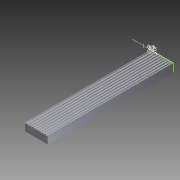
# Autodesk Inventor part: ruber2
Saved by Autodesk Inventor 2012 (Build 160160000, 160)
## iProperties
Created: 2013-08-22
Part Number: ruber2
Material: Default
Document SubType Name: Modeling
Designer: Dantro
Density: 1 g/cm^3
Author: Dantro
Autodesk Inventor part; units mm, degrees
ref_plane "YZ Plane" through (0, 0, 0) normal (1, 0, 0) x (0, 1, 0)
ref_plane "XZ Plane" through (0, 0, 0) normal (0, 1, 0) x (-1, 0, 0)
ref_plane "XY Plane" through (0, 0, 0) normal (0, 0, 1) x (1, 0, 0)
sketch "Sketch1" plane through (0, 0, 0) normal (0, 0, 1) x (1, 0, 0)
  line L0 (0, 0) -> (9, 0)
  line L1 (0.25, 3) -> (0, 3)
  line L2 (0.75, 3) -> (0.75, 2.7)
  line L3 (0.75, 2.7) -> (0.25, 2.7)
  line L4 (0.25, 2.7) -> (0.25, 3)
  line L5 (0.75, 3) -> (1, 3)
  line L6 (1.25, 3) -> (1, 3)
  line L7 (1.75, 3) -> (1.75, 2.7)
  line L8 (1.75, 2.7) -> (1.25, 2.7)
  line L9 (1.25, 2.7) -> (1.25, 3)
  line L10 (1.75, 3) -> (2, 3)
  line L11 (2.25, 3) -> (2, 3)
  line L12 (2.75, 3) -> (2.75, 2.7)
  line L13 (2.75, 2.7) -> (2.25, 2.7)
  line L14 (2.25, 2.7) -> (2.25, 3)
  line L15 (2.75, 3) -> (3, 3)
  line L16 (3.25, 3) -> (3, 3)
  line L17 (3.75, 3) -> (3.75, 2.7)
  line L18 (3.75, 2.7) -> (3.25, 2.7)
  line L19 (3.25, 2.7) -> (3.25, 3)
  line L20 (3.75, 3) -> (4, 3)
  line L21 (4.25, 3) -> (4, 3)
  line L22 (4.75, 3) -> (4.75, 2.7)
  line L23 (4.75, 2.7) -> (4.25, 2.7)
  line L24 (4.25, 2.7) -> (4.25, 3)
  line L25 (4.75, 3) -> (5, 3)
  line L26 (5.25, 3) -> (5, 3)
  line L27 (5.75, 3) -> (5.75, 2.7)
  line L28 (5.75, 2.7) -> (5.25, 2.7)
  line L29 (5.25, 2.7) -> (5.25, 3)
  line L30 (5.75, 3) -> (6, 3)
  line L31 (6.25, 3) -> (6, 3)
  line L32 (6.75, 3) -> (6.75, 2.7)
  line L33 (6.75, 2.7) -> (6.25, 2.7)
  line L34 (6.25, 2.7) -> (6.25, 3)
  line L35 (6.75, 3) -> (7, 3)
  line L36 (7.25, 3) -> (7, 3)
  line L37 (7.75, 3) -> (7.75, 2.7)
  line L38 (7.75, 2.7) -> (7.25, 2.7)
  line L39 (7.25, 2.7) -> (7.25, 3)
  line L40 (7.75, 3) -> (8, 3)
  line L41 (8.25, 3) -> (8, 3)
  line L42 (8.75, 3) -> (8.75, 2.7)
  line L43 (8.75, 2.7) -> (8.25, 2.7)
  line L44 (8.25, 2.7) -> (8.25, 3)
  line L45 (8.75, 3) -> (9, 3)
  line L46 (0, 3) -> (0, 0)
  line L47 (9, 3) -> (9, 0)
  dimension "d6" = 0.25
  dimension "d7" = 0.3
  dimension "d8" = 0.25
  dimension "d9" = 0.5
  dimension "d15" = 1
  constraints: 96 end point, 3 parallel, 2 horizontal, 2 perpendicular, 88 other
  measures "d6" distance of L1.start L1.end
  measures "d7" distance between parallel lines of L3 L1
  measures "d8" distance of L2.start L5.end
  measures "d9" distance of L2.end L3.end
  measures "d15" distance of L1.start L6.start
sketch "Sketch2" plane through (0, 0, 0) normal (0, 0, 1) x (1, 0, 0)
  line L0 (0, 0) -> (9, 0) projected
  line L1 (9, 3) -> (9, 0) projected
  line L2 (8.75, 3) -> (9, 3) projected
  line L3 (8.75, 3) -> (8.75, 2.7) projected
  line L4 (8.75, 2.7) -> (8.25, 2.7) projected
  line L5 (8.25, 2.7) -> (8.25, 3) projected
  line L6 (8.25, 3) -> (8, 3) projected
  line L7 (7.75, 3) -> (8, 3) projected
  line L8 (7.75, 3) -> (7.75, 2.7) projected
  line L9 (7.75, 2.7) -> (7.25, 2.7) projected
  line L10 (7.25, 2.7) -> (7.25, 3) projected
  line L11 (7.25, 3) -> (7, 3) projected
  line L12 (6.75, 3) -> (7, 3) projected
  line L13 (6.75, 3) -> (6.75, 2.7) projected
  line L14 (6.75, 2.7) -> (6.25, 2.7) projected
  line L15 (6.25, 2.7) -> (6.25, 3) projected
  line L16 (6.25, 3) -> (6, 3) projected
  line L17 (5.75, 3) -> (6, 3) projected
  line L18 (5.75, 3) -> (5.75, 2.7) projected
  line L19 (5.75, 2.7) -> (5.25, 2.7) projected
  line L20 (5.25, 2.7) -> (5.25, 3) projected
  line L21 (5.25, 3) -> (5, 3) projected
  line L22 (4.75, 3) -> (5, 3) projected
  line L23 (4.75, 3) -> (4.75, 2.7) projected
  line L24 (4.75, 2.7) -> (4.25, 2.7) projected
  line L25 (4.25, 2.7) -> (4.25, 3) projected
  line L26 (4.25, 3) -> (4, 3) projected
  line L27 (3.75, 3) -> (4, 3) projected
  line L28 (3.75, 3) -> (3.75, 2.7) projected
  line L29 (3.75, 2.7) -> (3.25, 2.7) projected
  line L30 (3.25, 2.7) -> (3.25, 3) projected
  line L31 (3.25, 3) -> (3, 3) projected
  line L32 (2.75, 3) -> (3, 3) projected
  line L33 (2.75, 3) -> (2.75, 2.7) projected
  line L34 (2.75, 2.7) -> (2.25, 2.7) projected
  line L35 (2.25, 2.7) -> (2.25, 3) projected
  line L36 (2.25, 3) -> (2, 3) projected
  line L37 (1.75, 3) -> (2, 3) projected
  line L38 (1.75, 3) -> (1.75, 2.7) projected
  line L39 (1.75, 2.7) -> (1.25, 2.7) projected
  line L40 (1.25, 2.7) -> (1.25, 3) projected
  line L41 (1.25, 3) -> (1, 3) projected
  line L42 (0.75, 3) -> (1, 3) projected
  line L43 (0.75, 3) -> (0.75, 2.7) projected
  line L44 (0.75, 2.7) -> (0.25, 2.7) projected
  line L45 (0.25, 2.7) -> (0.25, 3) projected
  line L46 (0.25, 3) -> (0, 3) projected
  line L47 (0, 3) -> (0, 0) projected
extrude "Extrusion1" add sketch "Sketch2" along normal blind 50
body "Solid1"
